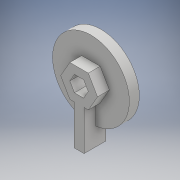
# Autodesk Inventor part: wingnut
Saved by Autodesk Inventor 2018 (Build 220112000, 112)
## iProperties
Created: 2017-10-25
Part Number: wingnut
Material: Generic
Document SubType Name: Modeling
Designer: Payal Jindal
Density: 1 g/cm^3
Appearance: Default
Author: Payal Jindal
Autodesk Inventor part; units mm, degrees
ref_plane "YZ Plane" through (0, 0, 0) normal (1, 0, 0) x (0, 1, 0)
ref_plane "XZ Plane" through (0, 0, 0) normal (0, 1, 0) x (-1, 0, 0)
ref_plane "XY Plane" through (0, 0, 0) normal (0, 0, 1) x (1, 0, 0)
sketch "Sketch1" plane through (0, 0, 0) normal (0, 1, 0) x (-1, 0, 0)
  line L0 (2.3094, 4) -> (4.6188, 0)
  line L1 (4.6188, 0) -> (2.3094, -4)
  line L2 (2.3094, -4) -> (-2.3094, -4)
  line L3 (-2.3094, -4) -> (-4.6188, 0)
  line L4 (-4.6188, 0) -> (-2.3094, 4)
  line L5 (-2.3094, 4) -> (2.3094, 4)
  line L6 (4.6188, -8) -> (9.2376, 0)
  line L7 (9.2376, 0) -> (4.6188, 8)
  line L8 (4.6188, 8) -> (-4.6188, 8)
  line L9 (-4.6188, 8) -> (-9.2376, 0)
  line L10 (-9.2376, 0) -> (-4.6188, -8)
  line L11 (-4.6188, -8) -> (4.6188, -8)
  point P0 (0, 0)
  point P1 (0, 0)
  dimension "d1" = 8
  dimension "d2" = 4
  constraints: 24 end point, 1 coincident, 1 horizontal, 18 other
  measures "d1" distance between parallel lines of L3 L0
  measures "d2" distance between parallel lines of L6 L1
extrude "Extrusion1" add sketch "Sketch1" along normal blind 5.9531
sketch "Sketch2" plane through (0, 5.9531, 0) normal (0, 1, 0) x (1, 0, 0)
  circle A0 centre (0, 0) radius 19.2376
  line L0 (4.6188, -8) -> (9.2376, 0) projected
  circle A1 centre (0, 0) radius 9.2376
  dimension "d5" = 10
  constraints: 2 coincident, 1 centre point, 1 horizontal alignment, 2 other
extrude "Extrusion2" add sketch "Sketch2" along normal blind 5 contours A0 | A1 L0 | L0 A1
sketch "Sketch3" plane through (0, 0, 0) normal (0, -1, 0) x (1, 0, 0)
  line L0 (4.6188, -8) -> (-4.6188, -8) projected
  line L1 (0, -8) -> (2.5, -8)
  line L2 (0, -8) -> (-2.5, -8)
  line L3 (2.5, -8) -> (-2.5, -8)
  line L4 (-2.5, -8) -> (-2.5, -28)
  line L5 (-2.5, -28) -> (2.5, -28)
  line L6 (2.5, -28) -> (2.5, -8)
  point P0 (0, 0)
  dimension "d8" = 2.5
  dimension "d9" = 2.5
  dimension "d10" = 20
  constraints: 12 end point, 2 parallel, 2 point on line, 1 horizontal, 1 midpoint, 1 perpendicular
  measures "d8" distance of L1.start L1.end
  measures "d9" distance of L1.start L2.end
  measures "d10" distance of L5.end L1.end
extrude "Extrusion3" add sketch "Sketch3" against normal up to surface (10.9531 mm away)
body "Solid1"
